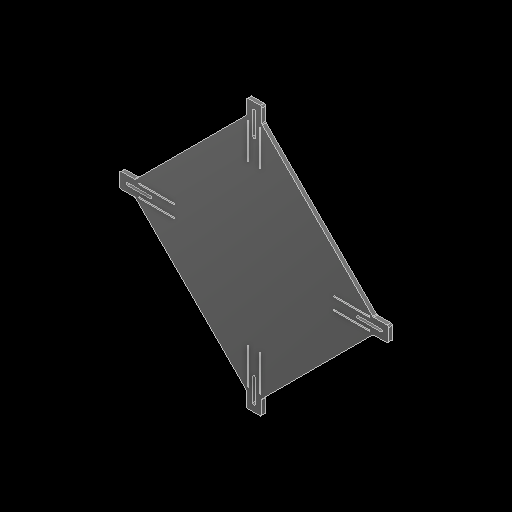
# Autodesk Inventor part: base_plate
Saved by Autodesk Inventor 2026.1 (Build 301233000, 233)
## iProperties
Created: 2025-09-14
Part Number: base_plate
Material: Aluminum 6061
Document SubType Name: Modeling
Designer: drago
Density: 2.7 g/cm^3
Appearance: Smooth - Black
Author: drago
Autodesk Inventor part; units mm, degrees
ref_plane "YZ Plane" through (0, 0, 0) normal (1, 0, 0) x (0, 1, 0)
ref_plane "XZ Plane" through (0, 0, 0) normal (0, 1, 0) x (-1, 0, 0)
ref_plane "XY Plane" through (0, 0, 0) normal (0, 0, 1) x (1, 0, 0)
sketch "Sketch2" plane through (0, 0, 0) normal (0, 0, 1) x (1, 0, 0)
  line L0 (307.5, 20) -> (347.5, 20)
  line L1 (347.5, 20) -> (347.5, -20)
  line L2 (347.5, -20) -> (307.5, -20)
  line L3 (307.5, -20) -> (307.5, 20)
  line L4 (307.5, 20) -> (347.5, -20) construction
  line L5 (347.5, 20) -> (307.5, -20) construction
  line L6 (327.5, 0) -> (-327.5, 0) construction
  line L7 (0, -327.5) -> (0, 327.5) construction
  line L8 (327.5, 0) -> (268.3955, 0) construction
  line L9 (327.5, 3.4) -> (268.3955, 3.4)
  line L10 (268.3955, -3.4) -> (327.5, -3.4)
  arc A0 (327.5, -3.4) -> (327.5, 3.4) centre (327.5, 0) ccw
  arc A1 (268.3955, 3.4) -> (268.3955, -3.4) centre (268.3955, 0) ccw
  line L11 (207.0955, 15.5) -> (297.2, 15.5) construction
  line L12 (207.0955, 13.9) -> (297.2, 13.9)
  line L13 (297.2, 17.1) -> (207.0955, 17.1)
  arc A2 (207.0955, 17.1) -> (207.0955, 13.9) centre (207.0955, 15.5) ccw
  arc A3 (297.2, 13.9) -> (297.2, 17.1) centre (297.2, 15.5) ccw
  line L14 (207.0955, -15.5) -> (297.2, -15.5) construction
  line L15 (207.0955, -17.1) -> (297.2, -17.1)
  line L16 (297.2, -13.9) -> (207.0955, -13.9)
  arc A4 (207.0955, -13.9) -> (207.0955, -17.1) centre (207.0955, -15.5) ccw
  arc A5 (297.2, -17.1) -> (297.2, -13.9) centre (297.2, -15.5) ccw
  arc A6 (-3.4, 268.3955) -> (3.4, 268.3955) centre (0, 268.3955) ccw
  line L17 (-13.9, 207.0955) -> (-13.9, 297.2)
  line L18 (-15.5, 207.0955) -> (-15.5, 297.2) construction
  line L19 (-17.1, 297.2) -> (-17.1, 207.0955)
  line L20 (17.1, 207.0955) -> (17.1, 297.2)
  line L21 (13.9, 297.2) -> (13.9, 207.0955)
  arc A7 (17.1, 297.2) -> (13.9, 297.2) centre (15.5, 297.2) ccw
  line L22 (20, 307.5) -> (-20, 307.5)
  line L23 (15.5, 207.0955) -> (15.5, 297.2) construction
  arc A8 (-17.1, 207.0955) -> (-13.9, 207.0955) centre (-15.5, 207.0955) ccw
  arc A9 (13.9, 207.0955) -> (17.1, 207.0955) centre (15.5, 207.0955) ccw
  line L24 (-20, 307.5) -> (-20, 347.5)
  line L25 (-20, 347.5) -> (20, 347.5)
  line L26 (20, 347.5) -> (20, 307.5)
  line L27 (-20, 307.5) -> (20, 347.5) construction
  line L28 (-20, 347.5) -> (20, 307.5) construction
  arc A10 (-13.9, 297.2) -> (-17.1, 297.2) centre (-15.5, 297.2) ccw
  line L29 (0, 327.5) -> (0, 268.3955) construction
  line L30 (3.4, 268.3955) -> (3.4, 327.5)
  arc A11 (3.4, 327.5) -> (-3.4, 327.5) centre (0, 327.5) ccw
  line L31 (-3.4, 327.5) -> (-3.4, 268.3955)
  arc A12 (-268.3955, -3.4) -> (-268.3955, 3.4) centre (-268.3955, 0) ccw
  line L32 (-207.0955, -13.9) -> (-297.2, -13.9)
  line L33 (-207.0955, -15.5) -> (-297.2, -15.5) construction
  line L34 (-297.2, -17.1) -> (-207.0955, -17.1)
  line L35 (-207.0955, 17.1) -> (-297.2, 17.1)
  line L36 (-297.2, 13.9) -> (-207.0955, 13.9)
  arc A13 (-297.2, 17.1) -> (-297.2, 13.9) centre (-297.2, 15.5) ccw
  line L37 (-307.5, 20) -> (-307.5, -20)
  line L38 (-207.0955, 15.5) -> (-297.2, 15.5) construction
  arc A14 (-207.0955, -17.1) -> (-207.0955, -13.9) centre (-207.0955, -15.5) ccw
  arc A15 (-207.0955, 13.9) -> (-207.0955, 17.1) centre (-207.0955, 15.5) ccw
  line L39 (-307.5, -20) -> (-347.5, -20)
  line L40 (-347.5, -20) -> (-347.5, 20)
  line L41 (-347.5, 20) -> (-307.5, 20)
  line L42 (-307.5, -20) -> (-347.5, 20) construction
  line L43 (-347.5, -20) -> (-307.5, 20) construction
  arc A16 (-297.2, -13.9) -> (-297.2, -17.1) centre (-297.2, -15.5) ccw
  line L44 (-327.5, 0) -> (-268.3955, 0) construction
  line L45 (-268.3955, 3.4) -> (-327.5, 3.4)
  arc A17 (-327.5, 3.4) -> (-327.5, -3.4) centre (-327.5, 0) ccw
  line L46 (-327.5, -3.4) -> (-268.3955, -3.4)
  arc A18 (3.4, -268.3955) -> (-3.4, -268.3955) centre (0, -268.3955) ccw
  line L47 (13.9, -207.0955) -> (13.9, -297.2)
  line L48 (15.5, -207.0955) -> (15.5, -297.2) construction
  line L49 (17.1, -297.2) -> (17.1, -207.0955)
  line L50 (-17.1, -207.0955) -> (-17.1, -297.2)
  line L51 (-13.9, -297.2) -> (-13.9, -207.0955)
  arc A19 (-17.1, -297.2) -> (-13.9, -297.2) centre (-15.5, -297.2) ccw
  line L52 (-20, -307.5) -> (20, -307.5)
  line L53 (-15.5, -207.0955) -> (-15.5, -297.2) construction
  arc A20 (17.1, -207.0955) -> (13.9, -207.0955) centre (15.5, -207.0955) ccw
  arc A21 (-13.9, -207.0955) -> (-17.1, -207.0955) centre (-15.5, -207.0955) ccw
  line L54 (20, -307.5) -> (20, -347.5)
  line L55 (20, -347.5) -> (-20, -347.5)
  line L56 (-20, -347.5) -> (-20, -307.5)
  line L57 (20, -307.5) -> (-20, -347.5) construction
  line L58 (20, -347.5) -> (-20, -307.5) construction
  arc A22 (13.9, -297.2) -> (17.1, -297.2) centre (15.5, -297.2) ccw
  line L59 (0, -327.5) -> (0, -268.3955) construction
  line L60 (-3.4, -268.3955) -> (-3.4, -327.5)
  arc A23 (-3.4, -327.5) -> (3.4, -327.5) centre (0, -327.5) ccw
  line L61 (3.4, -327.5) -> (3.4, -268.3955)
  line L62 (-307.5, 20) -> (-20, 307.5)
  line L63 (20, 307.5) -> (307.5, 20)
  line L64 (307.5, -20) -> (20, -307.5)
  line L65 (-20, -307.5) -> (-307.5, -20)
  point P0 (0, 0)
  point P1 (297.9478, 0)
  point P2 (252.1478, 15.5)
  point P3 (252.1478, -15.5)
  point P4 (15.5, 252.1478)
  point P5 (-15.5, 252.1478)
  point P6 (0, 297.9478)
  point P7 (-252.1478, 15.5)
  point P8 (-252.1478, -15.5)
  point P9 (-297.9478, 0)
  point P10 (-15.5, -252.1478)
  point P11 (15.5, -252.1478)
  point P12 (0, -297.9478)
  dimension "d148" = 40
  dimension "d149" = 655
  dimension "d154" = 59.1045
  dimension "d155" = 6.8
  dimension "d156" = 90.1045
  dimension "d157" = 3.2
  dimension "d171" = 31
  dimension "d172" = 10.3
  dimension "d173" = 10.3
  dimension "d176" = 360
  constraints: 156 end point, 48 point on circle, 24 centre point, 12 tangent, 7 midpoint, 5 parallel, 4 horizontal, 3 equal length, 3 perpendicular, 2 collinear, 1 equal radius, 1 point on line, 1 vertical, 187 other
  measures "d148" distance of L0.end L1.end
  measures "d149" distance of L6.start L6.end
  measures "d154" distance of L6.start L8.end
  measures "d155" diameter of A1
  measures "d156" distance of L11.start L11.end
  measures "d157" diameter of A3
  measures "d171" distance between parallel lines of L14 L11
  measures "d172" distance from line of L3 L11.end
  measures "d173" distance from line of L3 L14.end
extrude "Extrusion10" add sketch "Sketch2" against normal blind 10 contours L0 L1 L2 L3 L10 A0 L9 | L3 L9 A1 L10 L64 L52 L61 A18 L60 L65 L37 L46 A12 L45 L62 L22 L31 A6 L30 L63 | L22 L30 A11 L31 L24 L25 L26 | L54 L55 L56 L52 L60 A23 L61 | L37 L45 A17 L46 L39 L40 L41
fillet "Fillet8" radius 4 16 edges at (20, 347.5, -5) (-20, 347.5, -5) (-20, 307.5, -5) (-307.5, 20, -5) (-347.5, 20, -5) (-347.5, -20, -5) (347.5, 20, -5) (-20, -307.5, -5) (-20, -347.5, -5) (20, 307.5, -5) (20, -347.5, -5) (347.5, -20, -5) (307.5, -20, -5) (20, -307.5, -5) (307.5, 20, -5) (-307.5, -20, -5)
equation "\"ring_inner_diam\" = 565"
equation "\"ring_outer_diam\" = 615"
equation "\"dist_motor_bar\" = 10.3"
equation "\"motor_slot_diam\" = 3.2"
equation "\"motor_slot_length\" = 90.1045"
equation "\"bar_slot_diam\" = 6.8"
equation "\"bar_slot_length\" = 59.1045"
equation "\"dist_motor_holes\" = 31"
equation "\"diag_dist_bar_holes_old_fridge\" = 536.791"
equation "\"motor_dist_slots\" = 31"
equation "\"d162\" = 31"
equation "\"d163\" = 59.1045"
equation "\"d164\" = 536.791"
equation "\"d165\" = 615"
equation "\"d167\" = 565"
body "Solid4"
